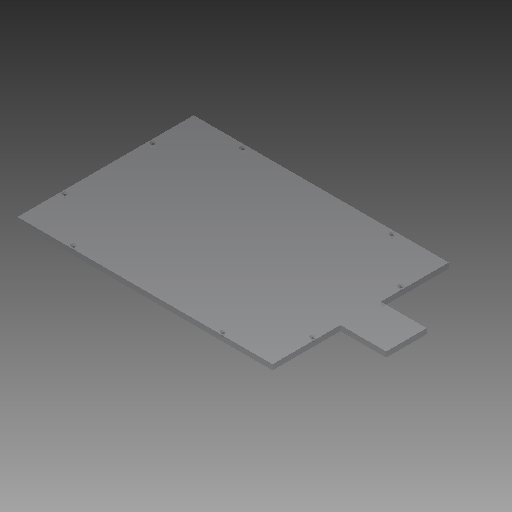
# Autodesk Inventor part: Deckel2
Saved by Autodesk Inventor 2018 (Build 220112000, 112)
## iProperties
Created: 2013-02-25
Part Number: Deckel2
Material: Polycarbonate, Clear
Document SubType Name: Modeling
Designer: Neef
Mass: 434.102 g
Surface Area: 1270.82 cm^2
Volume: 361.752 cm^3
Density: 1.2 g/cm^3
Appearance: Polycarbonate - Clear
Author: Neef
Autodesk Inventor part; units mm, degrees
ref_plane "YZ Plane" through (0, 0, 0) normal (1, 0, 0) x (0, 1, 0)
ref_plane "XZ Plane" through (0, 0, 0) normal (0, 1, 0) x (-1, 0, 0)
ref_plane "XY Plane" through (0, 0, 0) normal (0, 0, 1) x (1, 0, 0)
sketch "Skizze1" plane through (0, 0, 0) normal (0, 0, 1) x (1, 0, 0)
  line L0 (0, 120) -> (0, -20) projected
  line L1 (-68.3, 0) -> (409.8, 0) projected
  line L2 (0, 0) -> (217.779, 0)
  line L3 (289.5, 23) -> (289.5, 100)
  line L4 (289.5, 100) -> (0, 100)
  line L5 (0, 100) -> (0, 0)
  line L6 (217.779, 0) -> (341.5, 0)
  line L7 (341.5, 0) -> (341.5, 23)
  line L8 (341.5, 23) -> (289.5, 23)
  dimension "d0" = 52
  dimension "d1" = 289.5
  dimension "d2" = 100
  dimension "d3" = 23
  constraints: 14 end point, 3 parallel, 2 horizontal, 2 perpendicular
  measures "d0" distance of L7.end L3.start
  measures "d1" distance of L3.end L4.end
  measures "d2" distance of L4.end L2.start
  measures "d3" distance of L6.end L7.end
extrude "Extrusion1" add sketch "Skizze1" along normal blind 6
mirror "Spiegeln1" about plane through (217.779, 0, 0) normal (0, -1, 0)
sketch "Skizze2" plane through (0, 0, 6) normal (0, 0, 1) x (1, 0, 0)
  line L0 (0, -100) -> (0, 100) projected
  line L1 (289.5, 100) -> (289.5, 23) projected
  line L2 (0, 100) -> (289.5, 100) projected
  point P0 (0, 0)
  point P1 (60, 96)
  point P2 (229.5, 96)
  point P3 (4, 50)
  point P4 (285.5, 50)
  dimension "d6" = 60
  dimension "d7" = 60
  dimension "d8" = 50
  dimension "d9" = 50
  dimension "d10" = 4
  dimension "d11" = 4
  dimension "d12" = 4
  dimension "d13" = 4
  measures "d6" distance from line of L0 point (60, 96)
  measures "d7" distance from line of L1 point (229.5, 96)
  measures "d8" distance from line of L2 point (4, 50)
  measures "d9" distance from line of L2 point (285.5, 50)
  measures "d10" distance from line of L0 point (4, 50)
  measures "d11" distance from line of L2 point (60, 96)
  measures "d12" distance from line of L2 point (229.5, 96)
  measures "d13" distance from line of L1 point (285.5, 50)
hole "Bohrung1" at (60, 96, 6) at (229.5, 96, 6) at (4, 50, 6) at (285.5, 50, 6) direction (0, 0, -1) diameter 3.2 end through all countersink diameter 6.2 countersink angle 90
mirror "Spiegeln2" about plane through (0, 0, 0) normal (0, 1, 0) of "Bohrung1"
equation "\"d7\" = d6"
equation "\"d11\" = d10"
equation "\"d12\" = d11"
equation "\"d13\" = d12"
